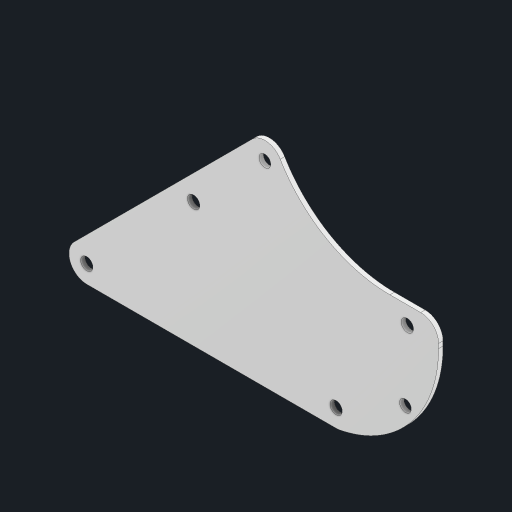
# Autodesk Inventor part: sled
Saved by Autodesk Inventor 2024 (Build 280153000, 153)
## iProperties
Created: 2023-08-16
Part Number: sled
Material: Acetal Resin, White
Document SubType Name: Modeling
Designer: avere
Density: 1.425 g/cm^3
Appearance: Smooth - White
Author: avere
Autodesk Inventor part; units mm, degrees
ref_plane "YZ Plane" through (0, 0, 0) normal (1, 0, 0) x (0, 1, 0)
ref_plane "XZ Plane" through (0, 0, 0) normal (0, 1, 0) x (-1, 0, 0)
ref_plane "XY Plane" through (0, 0, 0) normal (0, 0, 1) x (1, 0, 0)
sketch "Sketch1" plane through (0, 0, 0) normal (0, 0, 1) x (1, 0, 0)
  circle A0 centre (-18.372138, 25.147716) radius 2.1844
  circle A1 centre (57.827862, 25.147716) radius 2.1844
  circle A2 centre (32.427862, -12.952284) radius 2.1844
  circle A3 centre (-56.472138, -12.952284) radius 2.1844
  arc A4 (-60.962266, -8.462156) -> (-56.472138, -19.302284) centre (-56.472138, -12.952284) ccw
  arc A5 (-18.372138, 31.497716) -> (-22.862266, 29.637844) centre (-18.372138, 25.147716) ccw
  arc A6 (32.427862, -19.302284) -> (33.618646, -19.189634) centre (32.427862, -12.952284) ccw
  arc A7 (33.618646, -19.189634) -> (68.940362, 23.513344) centre (25.466144, 23.513344) ccw
  line L0 (68.940362, 23.513344) -> (68.940362, 25.147716)
  line L1 (62.590362, 31.497716) -> (57.827862, 31.497716)
  arc A8 (68.940362, 25.147716) -> (62.590362, 31.497716) centre (62.590362, 25.147716) ccw
  line L2 (32.427862, -19.302284) -> (-56.472138, -19.302284)
  line L3 (-60.962266, -8.462156) -> (-22.862266, 29.637844)
  line L4 (-18.372138, 31.497716) -> (57.827862, 31.497716)
  point P0 (0, 0)
  dimension "d0" = 4.3688
  dimension "d1" = 12.7
  dimension "d2" = 12.7
  dimension "d3" = 12.7
  dimension "d4" = 6.35
  constraints: 10 end point, 10 point on circle, 9 centre point, 9 tangent, 3 coincident, 2 vertical, 1 horizontal, 3 other
  measures "d0" diameter of A1
  measures "d1" diameter of A4
  measures "d2" diameter of A5
  measures "d3" diameter of A6
  measures "d4" radius of A8
extrude "Extrusion1" add sketch "Sketch1" along normal blind 1.5875
sketch "Sketch2" plane through (0, 0, 1.5875) normal (0, 0, 1) x (1, 0, 0)
  circle A0 centre (57.15, 0) radius 2.0828
  point P0 (0, 0)
  dimension "d7" = 4.1656
  constraints: 1 centre point
  measures "d7" diameter of A0
extrude "Extrusion2" cut sketch "Sketch2" against normal blind 1.5875
sketch "Sketch3" plane through (57.827862, 25.147716, 1.5875) normal (0, 0, 1) x (1, 0, 0)
  circle A0 centre (-50.8, 25.4) radius 2.0828
  arc A1 (-45.337489, 28.63782) -> (-55.290128, 29.890128) centre (-50.8, 25.4) ccw
  line L0 (-80.690128, 4.490128) -> (-55.290128, 29.890128)
  arc A2 (-76.2, 6.35) -> (-80.690128, 4.490128) centre (-76.2, 0) ccw
  arc A3 (-45.337489, 28.63782) -> (-6.21782, 6.35) centre (-6.21782, 51.825409) ccw
  line L1 (4.7625, 6.35) -> (-76.2, 6.35)
  dimension "d17" = 4.1656
  constraints: 5 point on circle, 4 tangent, 3 centre point, 2 end point, 1 coincident, 1 point on line, 1 other
  measures "d17" diameter of A0
extrude "Extrusion4" add sketch "Sketch3" against normal blind 1.5875
body "Solid1"
